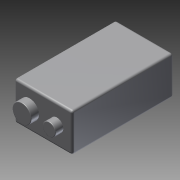
# Autodesk Inventor part: 276-2243
Saved by Autodesk Inventor 2013 (Build 170138000, 138)
## iProperties
Category: Power
Company: Autodesk Inc.
Created: 2012-02-07
Part Number: 276-2243
Document SubType Name: Modeling
Designer: Autodesk Inc.
Density: 1.06 g/cm^3
Material: ABS Plastic
Catalog Web Link: http://www.vexrobotics.com/276-2243.html
Vendor: VEX
Mass: 23.0526 g
Surface Area: 50.1473 cm^2
Volume: 21.7478 cm^3
Author: Autodesk Inc.
Autodesk Inventor part; units mm, degrees
ref_plane "YZ Plane" through (0, 0, 0) normal (1, 0, 0) x (0, 1, 0)
ref_plane "XZ Plane" through (0, 0, 0) normal (0, 1, 0) x (-1, 0, 0)
sketch "Sketch1" plane through (0, 0, 0) normal (0, 0, 1) x (1, 0, 0)
  line L0 (0, 0) -> (26.4922, 0)
  line L1 (26.4922, 0) -> (26.4922, 17.5006)
  line L2 (26.4922, 17.5006) -> (0, 17.5006)
  line L3 (0, 17.5006) -> (0, 0)
  dimension "d0" = 26.4922
  dimension "d1" = 17.5006
  constraints: 8 end point, 2 parallel, 1 horizontal, 1 perpendicular
  measures "d0" distance of L2.end L1.end
  measures "d1" distance of L0.end L1.end
extrude "Extrusion1" add sketch "Sketch1" against normal blind 46.4058
fillet "Fillet1" radius 0.9906 12 edges at (0, 17.5006, -23.2029) (0, 0, -23.2029) (0, 8.7503, 0) (0, 8.7503, -46.4058) (26.4922, 17.5006, -23.2029) (13.2461, 17.5006, 0) (13.2461, 17.5006, -46.4058) (26.4922, 0, -23.2029) (26.4922, 8.7503, 0) (26.4922, 8.7503, -46.4058) (13.2461, 0, 0) (13.2461, 0, -46.4058)
sketch "Sketch2" plane through (0, 0, 0) normal (0, 0, 1) x (1, 0, 0)
  line L0 (0.9906, 16.51) -> (25.5016, 16.51) projected
  line L1 (0.9906, 0.9906) -> (0.9906, 16.51) projected
  line L2 (0.9961, 16.5003) -> (25.4961, 16.5003)
  line L3 (0.9961, 16.5003) -> (0.9961, 1.0003)
  line L4 (0.9961, 1.0003) -> (25.4961, 1.0003)
  line L5 (25.4961, 1.0003) -> (25.4961, 16.5003)
  circle A0 centre (6.9961, 8.7503) radius 4.3
  circle A1 centre (19.4961, 8.7503) radius 2.95
  point P0 (0, 0)
  point P1 (13.2461, 8.7503)
  point P2 (13.2461, 8.7503)
  point P3 (13.2461, 16.51)
  point P4 (0.9906, 8.7503)
  constraints: 8 end point, 2 centre point, 2 midpoint, 1 horizontal alignment, 1 vertical alignment
extrude "Extrusion2" add sketch "Sketch2" along normal blind 3.6068 contours A0 | A1
fillet "Fillet2" radius 0.254 2 edges at (2.6961, 8.7503, 3.6068) (16.5461, 8.7503, 3.6068)
ref_plane "Work Plane1" through (13.2461, 0.9906, -45.4152) normal (1, 0, 0) x (0, 0, -1)
body "Solid1"
